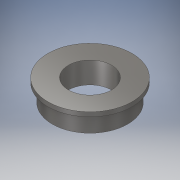
# Autodesk Inventor part: MF148ZZ
Saved by Autodesk Inventor 2019.4 (Build 234330000, 330)
## iProperties
Created: 2020-01-27
Part Number: MF148ZZ
Material: Steel, Mild
Document SubType Name: Modeling
Designer: admin
Density: 7.85 g/cm^3
Appearance: Semi-Polished
Author: admin
Autodesk Inventor part; units mm, degrees
ref_plane "YZ Plane" through (0, 0, 0) normal (1, 0, 0) x (0, 1, 0)
ref_plane "XZ Plane" through (0, 0, 0) normal (0, 1, 0) x (-1, 0, 0)
ref_plane "XY Plane" through (0, 0, 0) normal (0, 0, 1) x (1, 0, 0)
sketch "Sketch1" plane through (0, 0, 0) normal (0, 0, 1) x (1, 0, 0)
  line L0 (-4, 0) -> (-4, 4)
  line L1 (-4, 4) -> (-7.8, 4)
  line L2 (-7.8, 4) -> (-7.8, 3.2)
  line L3 (-7.8, 3.2) -> (-7, 3.2)
  line L4 (-7, 3.2) -> (-7, 0)
  line L5 (-7, 0) -> (-4, 0)
  line L6 (0, 0) -> (0, 3.606) construction
  dimension "d0" = 7.8
  dimension "d1" = 4
  dimension "d2" = 4
  dimension "d4" = 0.8
  dimension "d5" = 7
  constraints: 14 end point, 5 perpendicular, 2 vertical, 1 point on line
  measures "d0" distance between parallel lines of L6 L2
  measures "d1" distance between parallel lines of L6 L0
  measures "d2" distance of L0.start L0.end
  measures "d4" distance of L1.end L2.end
  measures "d5" distance between parallel lines of L6 L4
revolve "Revolution1" add sketch "Sketch1" angle 360 about axis through (0, 0, 0) along (0, 1, 0)
body "Solid1"
